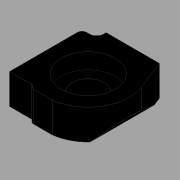
# Autodesk Inventor part: PocketNC_Workpiece_Z_axis_rotation
Saved by Autodesk Inventor 2017 (Build 210142000, 142)
## iProperties
Created: 2018-06-06
Part Number: PocketNC_Workpiece_Z_axis_rotation
Material: Generic
Document SubType Name: Modeling
Designer: Jarrett
Density: 1 g/cm^3
Appearance: Anodized - Black
Author: Jarrett
Autodesk Inventor part; units mm, degrees
ref_plane "YZ Plane" through (0, 0, 0) normal (1, 0, 0) x (0, 1, 0)
ref_plane "XZ Plane" through (0, 0, 0) normal (0, 1, 0) x (-1, 0, 0)
ref_plane "XY Plane" through (0, 0, 0) normal (0, 0, 1) x (1, 0, 0)
sketch "Sketch1" plane through (0, 0, 0) normal (0, 1, 0) x (-1, 0, 0)
  circle A0 centre (0, 0) radius 26.6
  line L0 (0, -26.6) -> (0, -74.6) construction
  line L1 (-44.5, -74.6) -> (44.5, -74.6)
  line L2 (0, 26.6) -> (0, 68.1) construction
  line L3 (-44.5, -74.6) -> (-63.8947, -24.9684)
  line L4 (26.6, 0) -> (69.1, 0) construction
  arc A1 (-8.2674, 68.1) -> (-63.8947, -24.9684) centre (0, 0) ccw
  line L5 (44.5, -74.6) -> (44.5, -70.6)
  line L6 (56.5, -58.6) -> (60.923, -58.6)
  arc A2 (56.5, -58.6) -> (44.5, -70.6) centre (56.5, -70.6) ccw
  arc A3 (60.923, -58.6) -> (68.923, -50.6) centre (60.923, -50.6) ccw
  line L7 (68.923, 68.1) -> (27.423, 68.1) construction
  line L8 (27.423, 68.1) -> (27.423, 62.6) construction
  line L9 (31.423, 62.6) -> (68.923, 62.6)
  line L10 (-8.2674, 68.1) -> (23.923, 68.1)
  line L11 (27.423, 66.6) -> (27.423, 64.6)
  line L12 (68.923, 62.6) -> (68.923, -50.6)
  arc A4 (27.423, 64.6) -> (23.923, 68.1) centre (23.923, 64.6) ccw
  arc A5 (27.423, 66.6) -> (31.423, 62.6) centre (31.423, 66.6) ccw
  point P0 (44.5, -58.6)
  dimension "d0" = 53.2
  dimension "d2" = 48
  dimension "d3" = 44.5
  dimension "d4" = 89
  dimension "d5" = 41.5
  dimension "d6" = 42.5
  dimension "d7" = 16
  dimension "d8" = 12
  dimension "d9" = 8
  dimension "d10" = 5.5
  dimension "d11" = 41.5
  dimension "d12" = 3.5
  dimension "d13" = 4
  constraints: 26 end point, 13 point on circle, 8 tangent, 6 centre point, 6 point on line, 3 horizontal, 3 vertical, 2 coincident, 2 perpendicular, 1 parallel
  measures "d0" diameter of A0
  measures "d2" distance of L0.start L0.end
  measures "d3" distance of L0.end L1.start
  measures "d4" distance of L1.start L1.end
  measures "d5" distance of L2.start L2.end
  measures "d6" distance of L4.start L4.end
  measures "d7" distance of L1.end point (44.5, -58.6)
  measures "d8" radius of A2
  measures "d9" radius of A3
  measures "d10" distance of L7.start L9.end
  measures "d11" distance of L7.start L7.end
  measures "d12" radius of A4
  measures "d13" radius of A5
extrude "Extrusion1" add sketch "Sketch1" along normal blind 50.5
sketch "Sketch2" plane through (0, 50.5, 0) normal (0, 1, 0) x (1, 0, 0)
  circle A0 centre (0, 0) radius 45
  dimension "d16" = 90
  constraints: 1 centre point, 1 coincident
  measures "d16" diameter of A0
extrude "Extrusion2" cut sketch "Sketch2" against normal blind 26
sketch "Sketch3" plane through (0, 0, 0) normal (0, 0, 1) x (1, 0, 0)
  line L0 (68.6, 22.5) -> (85.1798, 22.5)
  line L1 (68.6, 0) -> (50.1, 0)
  line L2 (68.6, 0) -> (8.2674, 0) projected
  line L3 (50.1, 0) -> (68.6, 22.5)
  line L4 (68.6, 0) -> (85.1798, 22.5)
  point P0 (0, 0)
  point P1 (63.8947, 0)
  dimension "d20" = 18.5
  constraints: 8 end point, 1 point on line
  measures "d20" distance of L1.start L1.end
extrude "Extrusion3" cut sketch "Sketch3" along normal mid plane 150
body "Solid1"
